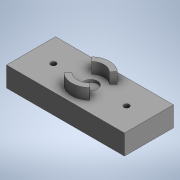
# Autodesk Inventor part: MG996R Arm Test
Saved by Autodesk Inventor 2020.5 (Build 245400000, 400)
## iProperties
Created: 2023-03-16
Part Number: MG996R Arm Test
Material: Generic
Document SubType Name: Modeling
Designer: Wes
Density: 1 g/cm^3
Appearance: Default
Author: Wes
Autodesk Inventor part; units mm, degrees
ref_plane "YZ Plane" through (0, 0, 0) normal (1, 0, 0) x (0, 1, 0)
ref_plane "XZ Plane" through (0, 0, 0) normal (0, 1, 0) x (-1, 0, 0)
ref_plane "XY Plane" through (0, 0, 0) normal (0, 0, 1) x (1, 0, 0)
sketch "Base" plane through (0, 0, 0) normal (0, 0, 1) x (1, 0, 0)
  line L0 (0, 0) -> (-22, 0)
  line L1 (-22, 0) -> (-22, 53)
  line L2 (-22, 53) -> (0, 53)
  line L3 (0, 53) -> (0, 0)
  line L4 (-11, 26.5) -> (-11, 43.6) construction
  line L5 (-11, 26.5) -> (-11, 9.4) construction
  line L6 (-11, 26.5) -> (-11, 10.7) construction
  line L7 (-11, 26.5) -> (-11, 42.3) construction
  line L8 (-11, 10.7) -> (-11, 9.4) construction
  line L9 (-11, 42.3) -> (-11, 43.6) construction
  circle A0 centre (-11, 42.95) radius 1.175
  circle A1 centre (-11, 10.05) radius 1.175
  dimension "d0" = 22
  dimension "d1" = 53
  dimension "d8" = 34.2
  dimension "d14" = 31.6
  dimension "d15" = 2.35
  dimension "d16" = 2.35
  constraints: 20 end point, 3 vertical, 2 centre point, 2 midpoint, 2 parallel, 2 point on line, 1 collinear, 1 horizontal, 1 perpendicular
  measures "d0" distance of L1.end L2.end
  measures "d1" distance of L0.end L1.end
  measures "d8" distance of L4.end L5.end
  measures "d14" distance of L7.end L6.end
  measures "d15" diameter of A0
  measures "d16" diameter of A1
extrude "Extrusion1" add sketch "Base" along normal mid plane 9
sketch "Countersink Arm Screw Holes" plane through (0, 0, -4.5) normal (0, 0, -1) x (-1, 0, 0)
  circle A0 centre (11, 10.05) radius 1.175 projected
  circle A1 centre (11, 10.05) radius 2.7
  circle A2 centre (11, 42.95) radius 1.175 projected
  circle A3 centre (11, 42.95) radius 2.7
  point P0 (0, 0)
  dimension "d19" = 5.4
  dimension "d20" = 5.4
  constraints: 2 centre point, 2 coincident
  measures "d19" diameter of A1
  measures "d20" diameter of A3
extrude "Extrusion2" cut sketch "Countersink Arm Screw Holes" against normal blind 1.8 contours A0 | A1 | A2 | A3
sketch "Servo Axle Screw Countersink" plane through (0, 0, 4.5) normal (0, 0, 1) x (1, 0, 0)
  circle A0 centre (-11.0894, 26.7154) radius 3.1
  point P0 (0, 0)
  dimension "d23" = 6.2
  constraints: 1 centre point
  measures "d23" diameter of A0
extrude "Extrusion3" cut sketch "Servo Axle Screw Countersink" against normal blind 1.2
sketch "Servo Arm Center Fitting" plane through (0, 0, 4.5) normal (0, 0, 1) x (1, 0, 0)
  circle A0 centre (-11.0894, 26.7154) radius 5.975 construction
  line L0 (-6.6965, 22.6654) -> (-6.6965, 30.7654) construction
  line L1 (-6.6965, 22.6654) -> (-15.4824, 22.6654) construction
  line L2 (-15.4824, 22.6654) -> (-15.4824, 30.7654) construction
  arc A1 (-15.4824, 30.7654) -> (-15.4824, 22.6654) centre (-11.0894, 26.7154) ccw
  line L3 (-15.4824, 22.6654) -> (-17.3205, 20.9709)
  line L4 (-15.4824, 30.7654) -> (-17.3205, 32.46)
  arc A2 (-17.3205, 32.46) -> (-17.3205, 20.9709) centre (-11.0894, 26.7154) ccw
  line L5 (-11.0894, 16.0563) -> (-11.0894, 38.4048) construction
  arc A3 (-6.6965, 22.6654) -> (-6.6965, 30.7654) centre (-11.0894, 26.7154) ccw
  line L6 (-6.6965, 22.6654) -> (-4.8584, 20.9709)
  line L7 (-6.6965, 30.7654) -> (-4.8584, 32.46)
  arc A4 (-4.8584, 20.9709) -> (-4.8584, 32.46) centre (-11.0894, 26.7154) ccw
  point P0 (0, 0)
  dimension "d27" = 11.95
  dimension "d31" = 8.1
  dimension "d32" = 8.1
  dimension "d33" = 2.5
  dimension "d34" = 2.5
  constraints: 16 end point, 12 point on circle, 5 centre point, 2 line through centre, 2 symmetric about line, 2 vertical, 1 coincident, 1 concentric, 1 perpendicular, 2 other
  measures "d27" diameter of A0
  measures "d31" distance of L0.start L0.end
  measures "d32" distance of L1.end L2.end
  measures "d33" distance of L1.end L3.end
  measures "d34" distance of L2.end L4.end
extrude "Extrusion4" add sketch "Servo Arm Center Fitting" along normal blind 5
body "Solid1"
